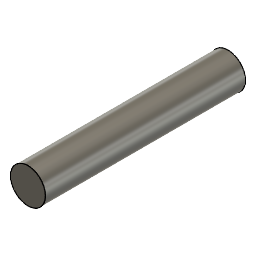
Assembly1 (Autodesk Fusion 360 archive; units mm, degrees)
design "attachment"
part number: 2026-09-06-17-01-46-998
Autodesk Fusion 360 part; units mm, degrees
sketch "Sketch1" plane through (0, 0, 0) normal (0, 0, 1) x (1, 0, 0)
  circle A0 centre (0, 0) radius 3.5
  dimension "d1" = 7
  constraint coincident A0.centre origin
  measures "d1" diameter of A0
extrude "Extrude1" add sketch "Sketch1" along normal blind 40
sketch "Sketch2" plane through (0, 0, 0) normal (0, 0, -1) x (-1, 0, 0)
  circle A0 centre (0, 0) radius 3.5
  circle A1 centre (0, 0) radius 3
  dimension "d4" = 6
  constraint concentric A0 A1
  measures "d4" diameter of A1
extrude "Extrude2" cut sketch "Sketch2" against normal blind 38 contours A1

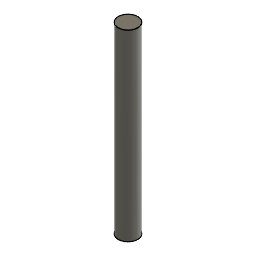
design "Leg"
part number: 2026-09-06-17-08-01-996
Autodesk Fusion 360 part; units mm, degrees
sketch "Sketch1" plane through (0, 0, 0) normal (0, 1, 0) x (1, 0, 0)
  circle A0 centre (0, 0) radius 3
  dimension "d1" = 6
  constraint coincident A0.centre origin
  measures "d1" diameter of A0
extrude "Extrude1" add sketch "Sketch1" along normal blind 56

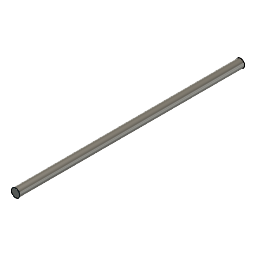
design "Tube1"
part number: 2026-09-06-16-51-40-034
Autodesk Fusion 360 part; units mm, degrees
sketch "Sketch1" plane through (0, 0, 0) normal (0, 0, 1) x (1, 0, 0)
  circle A0 centre (0, 0) radius 3
  dimension "d1" = 6
  constraint coincident A0.centre origin
  measures "d1" diameter of A0
extrude "Extrude1" add sketch "Sketch1" along normal blind 160
sketch "Sketch2" plane through (0, 0, 160) normal (0, 0, 1) x (1, 0, 0)
  circle A0 centre (0, 0) radius 3
